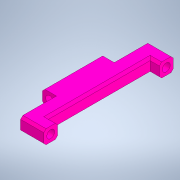
# Autodesk Inventor part: camadapter
Saved by Autodesk Inventor 2020 (Build 240168000, 168)
## iProperties
Created: 2020-11-07
Part Number: camadapter
Material: Generic
Document SubType Name: Modeling
Designer: alnwlsn
Density: 1 g/cm^3
Appearance: Default
Author: alnwlsn
Autodesk Inventor part; units mm, degrees
ref_plane "YZ Plane" through (0, 0, 0) normal (1, 0, 0) x (0, 1, 0)
ref_plane "XZ Plane" through (0, 0, 0) normal (0, 1, 0) x (-1, 0, 0)
ref_plane "XY Plane" through (0, 0, 0) normal (0, 0, 1) x (1, 0, 0)
sketch "Sketch1" plane through (0, 0, 0) normal (0, 1, 0) x (-1, 0, 0)
  line L0 (0, 0) -> (0, -6)
  line L1 (0, -6) -> (4, -6)
  line L2 (4, -6) -> (4, -50)
  line L3 (4, -50) -> (0, -50)
  line L4 (0, -50) -> (0, -56)
  line L5 (0, -56) -> (10, -56)
  line L6 (0, 0) -> (10, 0)
  line L7 (10, 0) -> (10, -15.5)
  line L8 (10, -15.5) -> (16, -15.5)
  line L9 (16, -40.5) -> (10, -40.5)
  line L10 (10, -40.5) -> (10, -56)
  line L11 (16, -15.5) -> (16, -40.5)
  point P0 (0, -3)
  point P1 (0, -53)
  dimension "d0" = 25
  dimension "d1" = 6
  dimension "d2" = 50
  dimension "d3" = 6
  dimension "d4" = 4
  dimension "d17" = 6
  constraints: 24 end point, 8 perpendicular, 3 equal length, 2 midpoint, 2 point on line, 2 vertical, 1 horizontal
  measures "d0" distance of L8.end L9.start
  measures "d1" distance of L7.end L8.end
  measures "d2" distance of point (0, -53) point (0, -3)
  measures "d3" distance between parallel lines of L6 L1
  measures "d4" distance between parallel lines of L0 L2
  measures "d17" distance between parallel lines of L2 L7
extrude "Extrusion1" add sketch "Sketch1" along normal blind 6
sketch "Sketch2" plane through (0, 0, 0) normal (1, 0, 0) x (0, 0, -1)
  line L0 (15.5, 6) -> (0, 6) projected
  line L1 (6, 0) -> (50, 0) projected
  line L2 (0, 6) -> (6, 0) construction
  line L3 (50, 0) -> (56, 0) projected
  line L4 (50, 0) -> (56, 6) construction
  circle A0 centre (3, 3) radius 1.7
  circle A1 centre (53, 3) radius 1.7
  point P0 (0, 0)
  dimension "d8" = 3.4
  constraints: 4 end point, 2 centre point, 2 midpoint, 1 equal radius, 1 perpendicular
  measures "d8" diameter of A0
extrude "Extrusion2" cut sketch "Sketch2" against normal through all
sketch "Sketch3" plane through (-16, 0, -15.5) normal (0, 0, 1) x (1, 0, 0)
  line L0 (16, 0) -> (6, 0) projected
  line L1 (0, 6) -> (6, 0) construction
  circle A0 centre (3, 3) radius 1.7
  dimension "d11" = 3.4
  constraints: 2 end point, 1 centre point, 1 midpoint
  measures "d11" diameter of A0
extrude "Extrusion3" cut sketch "Sketch3" against normal through all
chamfer "Chamfer1" distance 1 angle 45 12 edges at (-5, 6, 0) (-5, 0, 0) (-16, 6, -28) (-16, 0, -28) (-2, 6, -50) (-5, 6, -56) (-5, 0, -56) (-2, 0, -50) (-4, 6, -28) (-4, 0, -28) (-2, 6, -6) (-2, 0, -6)
equation "\"d3\" = d1"
equation "\"d6\" = d1"
body "Solid1"
